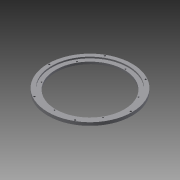
# Autodesk Inventor part: Turntable_2
Saved by Autodesk Inventor 2016 (Build 200138000, 138)
## iProperties
Created: 2016-04-11
Part Number: Turntable_2
Material: Generic
Document SubType Name: Modeling
Designer: rubenjm
Density: 1 g/cm^3
Appearance: Default
Author: rubenjm
Autodesk Inventor part; units mm, degrees
ref_plane "YZ Plane" through (0, 0, 0) normal (1, 0, 0) x (0, 1, 0)
ref_plane "XZ Plane" through (0, 0, 0) normal (0, 1, 0) x (-1, 0, 0)
ref_plane "XY Plane" through (0, 0, 0) normal (0, 0, 1) x (1, 0, 0)
sketch "Sketch1" plane through (0, 0, 0) normal (0, 1, 0) x (-1, 0, 0)
  circle A0 centre (0, 0) radius 162.56 construction
  circle A1 centre (0, 0) radius 148.0058
  circle A2 centre (0, 0) radius 132.461
  dimension "d0" = 325.12
  dimension "d1" = 296.0116
  dimension "d2" = 264.922
  constraints: 3 centre point, 3 coincident
  measures "d0" diameter of A0
  measures "d1" diameter of A1
  measures "d2" diameter of A2
extrude "Extrusion1" add sketch "Sketch1" along normal blind 1.778
sketch "Sketch2" plane through (0, 1.778, 0) normal (0, 1, 0) x (1, 0, 0)
  circle A0 centre (0, 0) radius 132.461
  circle A1 centre (0, 0) radius 162.56
  dimension "d5" = 325.12
  constraints: 2 centre point, 2 coincident
  measures "d5" diameter of A1
extrude "Extrusion2" add sketch "Sketch2" along normal blind 12.192
sketch "Sketch3" plane through (0, 13.97, 0) normal (0, 1, 0) x (1, 0, 0)
  circle A0 centre (0, 0) radius 148.0058
  circle A1 centre (0, 0) radius 132.461
  constraints: 2 centre point, 2 coincident
extrude "Extrusion3" cut sketch "Sketch3" against normal blind 5.588
sketch "Sketch4" plane through (0, 13.97, 0) normal (0, 1, 0) x (1, 0, 0)
  circle A0 centre (0, 0) radius 157.48 construction
  circle A1 centre (-157.48, 0) radius 3.9687
  circle A2 centre (-78.74, -136.3817) radius 3.9687
  circle A3 centre (78.74, -136.3817) radius 3.9687
  circle A4 centre (157.48, 0) radius 3.9687
  circle A5 centre (78.74, 136.3817) radius 3.9687
  circle A6 centre (-78.74, 136.3817) radius 3.9687
  dimension "d10" = 314.96
  dimension "d11" = 7.9375
  dimension "d14" = 360
  constraints: 6 centre point, 1 coincident, 1 horizontal alignment, 15 other
  measures "d11" diameter of A1
hole "Hole1" at (-157.48, 13.97, 0) at (78.74, 13.97, -136.3817) at (-78.74, 13.97, -136.3817) at (157.48, 13.97, 0) at (78.74, 13.97, 136.3817) at (-78.74, 13.97, 136.3817) direction (0, -1, 0) diameter 6.4008 depth 22.9362 thread size "5/16-18 UNC" class "2B" standard "ANSI Unified Screw Threads"
sketch "Sketch5" plane through (0, 8.382, 0) normal (0, 1, 0) x (1, 0, 0)
  line L0 (0, 0) -> (-122.3635, 70.6466) construction
  line L1 (0, 0) -> (141.2932, 0) construction
  line L2 (-122.3635, 70.6466) -> (0, 0) construction
  line L3 (0, 0) -> (-128.1768, -74.0029) construction
  circle A0 centre (0, 0) radius 148.0058 construction
  line L4 (0, 0) -> (148.0058, 0) construction
  circle A1 centre (0, 0) radius 137.541 construction
  circle A2 centre (-119.114, -68.7705) radius 3.175
  circle A3 centre (0, -137.541) radius 3.175
  circle A4 centre (119.114, -68.7705) radius 3.175
  circle A5 centre (119.114, 68.7705) radius 3.175
  circle A6 centre (0, 137.541) radius 3.175
  circle A7 centre (-119.114, 68.7705) radius 3.175
  dimension "d25" = 275.082
  dimension "d23" = 150
  dimension "d24" = 150
  dimension "d26" = 6.35
  dimension "d29" = 360
  constraints: 10 end point, 6 centre point, 2 equal length, 2 horizontal, 1 coincident, 1 collinear, 1 point on line, 18 other
  measures "d23" angle of L1 L0
  measures "d24" angle of L3 L4
  measures "d26" diameter of A2
hole "Hole2" at (0, 8.382, 137.541) at (119.114, 8.382, 68.7705) at (119.114, 8.382, -68.7705) at (0, 8.382, -137.541) at (-119.114, 8.382, -68.7705) at (-119.114, 8.382, 68.7705) direction (0, -1, 0) diameter 4.9784 depth 19.05 thread size "1/4-20 UNC" class "2B" standard "ANSI Unified Screw Threads"
body "Solid1"
